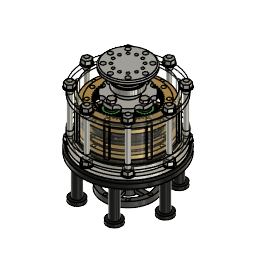
DualStagePlanetaryGearbox_2_5D_AI_Model (Autodesk Fusion 360 design; units mm, degrees)
part number: 2026-08-16-05-24-14-088
part number: 2026-08-16-14-10-31-109
part number: 2026-08-16-14-10-31-333
part number: 2026-08-16-14-11-30-504
part number: 2026-08-16-14-11-31-335
part number: 2026-08-16-14-11-32-044
part number: 2026-08-16-14-11-32-830
part number: 2026-08-16-14-11-50-183
part number: 2026-08-16-14-13-28-663
part number: 2026-08-16-14-13-28-868
part number: 2026-08-16-14-13-29-316
part number: 2026-08-16-14-13-29-716
part number: 2026-08-16-14-14-26-011
part number: 2026-08-16-14-14-26-279
part number: 2026-08-16-14-14-26-987
part number: 2026-08-16-14-14-27-816
part number: 2026-08-16-14-14-28-706
part number: 2026-08-16-14-14-29-780
part number: 2026-08-16-14-14-30-829
part number: 2026-08-16-14-16-16-341
part number: 2026-08-16-14-16-17-067
part number: 2026-08-16-14-16-17-350
part number: 2026-08-16-14-17-27-014
part number: 2026-08-16-14-17-28-983
part number: 2026-08-16-14-17-29-961
part number: 2026-08-16-14-17-30-254
part number: 2026-08-16-14-17-56-289
Autodesk Fusion 360 part; units mm, degrees
note: some values were not read from the file. Chosen so that the rebuilt part matches the saved one: which bodies a step acts on.
(part 1 of 5)
sketch "スケッチ1" plane through (0, 0, 0) normal (0, 0, 1) x (1, 0, 0) in component "Lower_Base_Plate"
  circle A0 centre (0, 0) radius 84
extrude "Base_Plate_Extrude" add sketch "スケッチ1" along normal blind 14 makes body 1 in component "Lower_Base_Plate"
sketch "スケッチ2" plane through (0, 0, 0) normal (0, 0, 1) x (1, 0, 0) in component "Lower_Base_Plate"
  circle A0 centre (0, 0) radius 32
extrude "Base_Center_Boss_Extrude" add sketch "スケッチ2" along normal blind 6 from surface at 14 bodies 1 in component "Lower_Base_Plate"
sketch "スケッチ3" plane through (0, 0, 0) normal (0, 0, 1) x (1, 0, 0) in component "Lower_Base_Plate"
  circle A0 centre (68, 0) radius 8
  circle A1 centre (34, 58.8897) radius 8
  circle A2 centre (-34, 58.8897) radius 8
  circle A3 centre (-68, 0) radius 8
  circle A4 centre (-34, -58.8897) radius 8
  circle A5 centre (34, -58.8897) radius 8
extrude "Base_Foot_Post_Extrude" add sketch "スケッチ3" along normal blind 56 from surface at -56 bodies 1 in component "Lower_Base_Plate"
sketch "スケッチ4" plane through (0, 0, 0) normal (0, 0, 1) x (1, 0, 0) in component "Lower_Base_Plate"
  circle A0 centre (68, 0) radius 13
  circle A1 centre (34, 58.8897) radius 13
  circle A2 centre (-34, 58.8897) radius 13
  circle A3 centre (-68, 0) radius 13
  circle A4 centre (-34, -58.8897) radius 13
  circle A5 centre (34, -58.8897) radius 13
extrude "Base_Foot_Pad_Extrude" add sketch "スケッチ4" along normal blind 6 from surface at -62 bodies 1 in component "Lower_Base_Plate"
sketch "スケッチ5" plane through (0, 0, 0) normal (0, 0, 1) x (1, 0, 0) in component "Lower_Base_Plate"
  circle A0 centre (0, 0) radius 13
extrude "Base_Center_Bore_Cut" cut sketch "スケッチ5" along normal blind 22 from surface at -1 bodies 1 in component "Lower_Base_Plate"
sketch "スケッチ6" plane through (0, 0, 0) normal (0, 0, 1) x (1, 0, 0) in component "Lower_Base_Plate"
  circle A0 centre (75, 0) radius 4.6
  circle A1 centre (53.033, 53.033) radius 4.6
  circle A2 centre (0, 75) radius 4.6
  circle A3 centre (-53.033, 53.033) radius 4.6
  circle A4 centre (-75, 0) radius 4.6
  circle A5 centre (-53.033, -53.033) radius 4.6
  circle A6 centre (0, -75) radius 4.6
  circle A7 centre (53.033, -53.033) radius 4.6
extrude "Base_TieRod_Hole_Cut" cut sketch "スケッチ6" along normal blind 16 from surface at -1 bodies 1 in component "Lower_Base_Plate"
sketch "スケッチ7" plane through (0, 0, 0) normal (0, 0, 1) x (1, 0, 0) in component "Lower_Base_Plate"
  circle A0 centre (48.0417, 19.8995) radius 9
  circle A1 centre (19.8995, 48.0417) radius 9
  circle A2 centre (-19.8995, 48.0417) radius 9
  circle A3 centre (-48.0417, 19.8995) radius 9
  circle A4 centre (-48.0417, -19.8995) radius 9
  circle A5 centre (-19.8995, -48.0417) radius 9
  circle A6 centre (19.8995, -48.0417) radius 9
  circle A7 centre (48.0417, -19.8995) radius 9
extrude "Base_Lightening_Hole_Cut" cut sketch "スケッチ7" along normal blind 16 from surface at -1 bodies 1 in component "Lower_Base_Plate"
sketch "スケッチ1 (2)" plane through (0, 0, 0) normal (0, 0, 1) x (1, 0, 0) in component "Lower_Housing_Ring"
  circle A0 centre (0, 0) radius 72
extrude "Housing_Ring_Extrude" add sketch "スケッチ1 (2)" along normal blind 16 from surface at 14 separate body makes body 2 in component "Lower_Housing_Ring"
sketch "スケッチ2 (2)" plane through (0, 0, 0) normal (0, 0, 1) x (1, 0, 0) in component "Lower_Housing_Ring"
  circle A0 centre (0, 0) radius 80
extrude "Housing_Ring_Flange_Extrude" add sketch "スケッチ2 (2)" along normal blind 6 from surface at 14 bodies 2 in component "Lower_Housing_Ring"
sketch "スケッチ3 (2)" plane through (0, 0, 0) normal (0, 0, 1) x (1, 0, 0) in component "Lower_Housing_Ring"
  circle A0 centre (0, 0) radius 64
extrude "Housing_Ring_Bore_Cut" cut sketch "スケッチ3 (2)" along normal blind 18 from surface at 13 bodies 2 in component "Lower_Housing_Ring"
sketch "スケッチ4 (2)" plane through (0, 0, 0) normal (0, 0, 1) x (1, 0, 0) in component "Lower_Housing_Ring"
  circle A0 centre (0, 0) radius 68
extrude "Housing_Ring_Top_Step_Cut" cut sketch "スケッチ4 (2)" along normal blind 4 from surface at 27 bodies 2 in component "Lower_Housing_Ring"
sketch "スケッチ5 (2)" plane through (0, 0, 0) normal (0, 0, 1) x (1, 0, 0) in component "Lower_Housing_Ring"
  circle A0 centre (75, 0) radius 4.6
  circle A1 centre (53.033, 53.033) radius 4.6
  circle A2 centre (0, 75) radius 4.6
  circle A3 centre (-53.033, 53.033) radius 4.6
  circle A4 centre (-75, 0) radius 4.6
  circle A5 centre (-53.033, -53.033) radius 4.6
  circle A6 centre (0, -75) radius 4.6
  circle A7 centre (53.033, -53.033) radius 4.6
extrude "Housing_Flange_Bolt_Hole_Cut" cut sketch "スケッチ5 (2)" along normal blind 8 from surface at 13 bodies 2 in component "Lower_Housing_Ring"
sketch "スケッチ1 (3)" plane through (0, 0, 0) normal (0, 0, 1) x (1, 0, 0) in component "Stage1_Sun_Gear"
  line L0 (16.0751, -1.2675) -> (16.8621, -1.3296)
  line L1 (16.8621, -1.3296) -> (17.7351, -1.2093)
  line L2 (17.7351, -1.2093) -> (18.6155, -0.9191)
  line L3 (18.6155, -0.9191) -> (19.4935, -0.5041)
  line L4 (19.4935, -0.5041) -> (19.4935, 0.5041)
  line L5 (19.4935, 0.5041) -> (18.6155, 0.9191)
  line L6 (18.6155, 0.9191) -> (17.7351, 1.2093)
  line L7 (17.7351, 1.2093) -> (16.8621, 1.3296)
  line L8 (16.8621, 1.3296) -> (16.0751, 1.2675)
  line L9 (16.0751, 1.2675) -> (15.987, 2.1047)
  line L10 (15.987, 2.1047) -> (15.8554, 2.9362)
  line L11 (15.8554, 2.9362) -> (16.6317, 3.08)
  line L12 (16.6317, 3.08) -> (17.4438, 3.422)
  line L13 (17.4438, 3.422) -> (18.2191, 3.9303)
  line L14 (18.2191, 3.9303) -> (18.9597, 4.5584)
  line L15 (18.9597, 4.5584) -> (18.6988, 5.5322)
  line L16 (18.6988, 5.5322) -> (17.7433, 5.7058)
  line L17 (17.7433, 5.7058) -> (16.8178, 5.7583)
  line L18 (16.8178, 5.7583) -> (15.9434, 5.6485)
  line L19 (15.9434, 5.6485) -> (15.1993, 5.3849)
  line L20 (15.1993, 5.3849) -> (14.8976, 6.1708)
  line L21 (14.8976, 6.1708) -> (14.5552, 6.9398)
  line L22 (14.5552, 6.9398) -> (15.2678, 7.2796)
  line L23 (15.2678, 7.2796) -> (15.9637, 7.8202)
  line L24 (15.9637, 7.8202) -> (16.581, 8.5118)
  line L25 (16.581, 8.5118) -> (17.1339, 9.3102)
  line L26 (17.1339, 9.3102) -> (16.6298, 10.1833)
  line L27 (16.6298, 10.1833) -> (15.6619, 10.1037)
  line L28 (15.6619, 10.1037) -> (14.7544, 9.9149)
  line L29 (14.7544, 9.9149) -> (13.9382, 9.5825)
  line L30 (13.9382, 9.5825) -> (13.2877, 9.1353)
  line L31 (13.2877, 9.1353) -> (12.7928, 9.8163)
  line L32 (12.7928, 9.8163) -> (12.2631, 10.4705)
  line L33 (12.2631, 10.4705) -> (12.8635, 10.9832)
  line L34 (12.8635, 10.9832) -> (13.3958, 11.6855)
  line L35 (13.3958, 11.6855) -> (13.813, 12.5132)
  line L36 (13.813, 12.5132) -> (14.1404, 13.4275)
  line L37 (14.1404, 13.4275) -> (13.4275, 14.1404)
  line L38 (13.4275, 14.1404) -> (12.5132, 13.813)
  line L39 (12.5132, 13.813) -> (11.6855, 13.3958)
  line L40 (11.6855, 13.3958) -> (10.9832, 12.8635)
  line L41 (10.9832, 12.8635) -> (10.4705, 12.2631)
  line L42 (10.4705, 12.2631) -> (9.8163, 12.7928)
  line L43 (9.8163, 12.7928) -> (9.1353, 13.2877)
  line L44 (9.1353, 13.2877) -> (9.5825, 13.9382)
  line L45 (9.5825, 13.9382) -> (9.9149, 14.7544)
  line L46 (9.9149, 14.7544) -> (10.1037, 15.6619)
  line L47 (10.1037, 15.6619) -> (10.1833, 16.6298)
  line L48 (10.1833, 16.6298) -> (9.3102, 17.1339)
  line L49 (9.3102, 17.1339) -> (8.5118, 16.581)
  line L50 (8.5118, 16.581) -> (7.8202, 15.9637)
  line L51 (7.8202, 15.9637) -> (7.2796, 15.2678)
  line L52 (7.2796, 15.2678) -> (6.9398, 14.5552)
  line L53 (6.9398, 14.5552) -> (6.1708, 14.8976)
  line L54 (6.1708, 14.8976) -> (5.3849, 15.1993)
  line L55 (5.3849, 15.1993) -> (5.6485, 15.9434)
  line L56 (5.6485, 15.9434) -> (5.7583, 16.8178)
  line L57 (5.7583, 16.8178) -> (5.7058, 17.7433)
  line L58 (5.7058, 17.7433) -> (5.5322, 18.6988)
  line L59 (5.5322, 18.6988) -> (4.5584, 18.9597)
  line L60 (4.5584, 18.9597) -> (3.9303, 18.2191)
  line L61 (3.9303, 18.2191) -> (3.422, 17.4438)
  line L62 (3.422, 17.4438) -> (3.08, 16.6317)
  line L63 (3.08, 16.6317) -> (2.9362, 15.8554)
  line L64 (2.9362, 15.8554) -> (2.1047, 15.987)
  line L65 (2.1047, 15.987) -> (1.2675, 16.0751)
  line L66 (1.2675, 16.0751) -> (1.3296, 16.8621)
  line L67 (1.3296, 16.8621) -> (1.2093, 17.7351)
  line L68 (1.2093, 17.7351) -> (0.9191, 18.6155)
  line L69 (0.9191, 18.6155) -> (0.5041, 19.4935)
  line L70 (0.5041, 19.4935) -> (-0.5041, 19.4935)
  line L71 (-0.5041, 19.4935) -> (-0.9191, 18.6155)
  line L72 (-0.9191, 18.6155) -> (-1.2093, 17.7351)
  line L73 (-1.2093, 17.7351) -> (-1.3296, 16.8621)
  line L74 (-1.3296, 16.8621) -> (-1.2675, 16.0751)
  line L75 (-1.2675, 16.0751) -> (-2.1047, 15.987)
  line L76 (-2.1047, 15.987) -> (-2.9362, 15.8554)
  line L77 (-2.9362, 15.8554) -> (-3.08, 16.6317)
  line L78 (-3.08, 16.6317) -> (-3.422, 17.4438)
  line L79 (-3.422, 17.4438) -> (-3.9303, 18.2191)
  line L80 (-3.9303, 18.2191) -> (-4.5584, 18.9597)
  line L81 (-4.5584, 18.9597) -> (-5.5322, 18.6988)
  line L82 (-5.5322, 18.6988) -> (-5.7058, 17.7433)
  line L83 (-5.7058, 17.7433) -> (-5.7583, 16.8178)
  line L84 (-5.7583, 16.8178) -> (-5.6485, 15.9434)
  line L85 (-5.6485, 15.9434) -> (-5.3849, 15.1993)
  line L86 (-5.3849, 15.1993) -> (-6.1708, 14.8976)
  line L87 (-6.1708, 14.8976) -> (-6.9398, 14.5552)
  line L88 (-6.9398, 14.5552) -> (-7.2796, 15.2678)
  line L89 (-7.2796, 15.2678) -> (-7.8202, 15.9637)
  line L90 (-7.8202, 15.9637) -> (-8.5118, 16.581)
  line L91 (-8.5118, 16.581) -> (-9.3102, 17.1339)
  line L92 (-9.3102, 17.1339) -> (-10.1833, 16.6298)
  line L93 (-10.1833, 16.6298) -> (-10.1037, 15.6619)
  line L94 (-10.1037, 15.6619) -> (-9.9149, 14.7544)
  line L95 (-9.9149, 14.7544) -> (-9.5825, 13.9382)
  line L96 (-9.5825, 13.9382) -> (-9.1353, 13.2877)
  line L97 (-9.1353, 13.2877) -> (-9.8163, 12.7928)
  line L98 (-9.8163, 12.7928) -> (-10.4705, 12.2631)
  line L99 (-10.4705, 12.2631) -> (-10.9832, 12.8635)
  line L100 (-10.9832, 12.8635) -> (-11.6855, 13.3958)
  line L101 (-11.6855, 13.3958) -> (-12.5132, 13.813)
  line L102 (-12.5132, 13.813) -> (-13.4275, 14.1404)
  line L103 (-13.4275, 14.1404) -> (-14.1404, 13.4275)
  line L104 (-14.1404, 13.4275) -> (-13.813, 12.5132)
  line L105 (-13.813, 12.5132) -> (-13.3958, 11.6855)
  line L106 (-13.3958, 11.6855) -> (-12.8635, 10.9832)
  line L107 (-12.8635, 10.9832) -> (-12.2631, 10.4705)
  line L108 (-12.2631, 10.4705) -> (-12.7928, 9.8163)
  line L109 (-12.7928, 9.8163) -> (-13.2877, 9.1353)
  line L110 (-13.2877, 9.1353) -> (-13.9382, 9.5825)
  line L111 (-13.9382, 9.5825) -> (-14.7544, 9.9149)
  line L112 (-14.7544, 9.9149) -> (-15.6619, 10.1037)
  line L113 (-15.6619, 10.1037) -> (-16.6298, 10.1833)
  line L114 (-16.6298, 10.1833) -> (-17.1339, 9.3102)
  line L115 (-17.1339, 9.3102) -> (-16.581, 8.5118)
  line L116 (-16.581, 8.5118) -> (-15.9637, 7.8202)
  line L117 (-15.9637, 7.8202) -> (-15.2678, 7.2796)
  line L118 (-15.2678, 7.2796) -> (-14.5552, 6.9398)
  line L119 (-14.5552, 6.9398) -> (-14.8976, 6.1708)
  line L120 (-14.8976, 6.1708) -> (-15.1993, 5.3849)
  line L121 (-15.1993, 5.3849) -> (-15.9434, 5.6485)
  line L122 (-15.9434, 5.6485) -> (-16.8178, 5.7583)
  line L123 (-16.8178, 5.7583) -> (-17.7433, 5.7058)
  line L124 (-17.7433, 5.7058) -> (-18.6988, 5.5322)
  line L125 (-18.6988, 5.5322) -> (-18.9597, 4.5584)
  line L126 (-18.9597, 4.5584) -> (-18.2191, 3.9303)
  line L127 (-18.2191, 3.9303) -> (-17.4438, 3.422)
  line L128 (-17.4438, 3.422) -> (-16.6317, 3.08)
  line L129 (-16.6317, 3.08) -> (-15.8554, 2.9362)
  line L130 (-15.8554, 2.9362) -> (-15.987, 2.1047)
  line L131 (-15.987, 2.1047) -> (-16.0751, 1.2675)
  line L132 (-16.0751, 1.2675) -> (-16.8621, 1.3296)
  line L133 (-16.8621, 1.3296) -> (-17.7351, 1.2093)
  line L134 (-17.7351, 1.2093) -> (-18.6155, 0.9191)
  line L135 (-18.6155, 0.9191) -> (-19.4935, 0.5041)
  line L136 (-19.4935, 0.5041) -> (-19.4935, -0.5041)
  line L137 (-19.4935, -0.5041) -> (-18.6155, -0.9191)
  line L138 (-18.6155, -0.9191) -> (-17.7351, -1.2093)
  line L139 (-17.7351, -1.2093) -> (-16.8621, -1.3296)
  line L140 (-16.8621, -1.3296) -> (-16.0751, -1.2675)
  line L141 (-16.0751, -1.2675) -> (-15.987, -2.1047)
  line L142 (-15.987, -2.1047) -> (-15.8554, -2.9362)
  line L143 (-15.8554, -2.9362) -> (-16.6317, -3.08)
  line L144 (-16.6317, -3.08) -> (-17.4438, -3.422)
  line L145 (-17.4438, -3.422) -> (-18.2191, -3.9303)
  line L146 (-18.2191, -3.9303) -> (-18.9597, -4.5584)
  line L147 (-18.9597, -4.5584) -> (-18.6988, -5.5322)
  line L148 (-18.6988, -5.5322) -> (-17.7433, -5.7058)
  line L149 (-17.7433, -5.7058) -> (-16.8178, -5.7583)
  line L150 (-16.8178, -5.7583) -> (-15.9434, -5.6485)
  line L151 (-15.9434, -5.6485) -> (-15.1993, -5.3849)
  line L152 (-15.1993, -5.3849) -> (-14.8976, -6.1708)
  line L153 (-14.8976, -6.1708) -> (-14.5552, -6.9398)
  line L154 (-14.5552, -6.9398) -> (-15.2678, -7.2796)
  line L155 (-15.2678, -7.2796) -> (-15.9637, -7.8202)
  line L156 (-15.9637, -7.8202) -> (-16.581, -8.5118)
  line L157 (-16.581, -8.5118) -> (-17.1339, -9.3102)
  line L158 (-17.1339, -9.3102) -> (-16.6298, -10.1833)
  line L159 (-16.6298, -10.1833) -> (-15.6619, -10.1037)
  line L160 (-15.6619, -10.1037) -> (-14.7544, -9.9149)
  line L161 (-14.7544, -9.9149) -> (-13.9382, -9.5825)
  line L162 (-13.9382, -9.5825) -> (-13.2877, -9.1353)
  line L163 (-13.2877, -9.1353) -> (-12.7928, -9.8163)
  line L164 (-12.7928, -9.8163) -> (-12.2631, -10.4705)
  line L165 (-12.2631, -10.4705) -> (-12.8635, -10.9832)
  line L166 (-12.8635, -10.9832) -> (-13.3958, -11.6855)
  line L167 (-13.3958, -11.6855) -> (-13.813, -12.5132)
  line L168 (-13.813, -12.5132) -> (-14.1404, -13.4275)
  line L169 (-14.1404, -13.4275) -> (-13.4275, -14.1404)
  line L170 (-13.4275, -14.1404) -> (-12.5132, -13.813)
  line L171 (-12.5132, -13.813) -> (-11.6855, -13.3958)
  line L172 (-11.6855, -13.3958) -> (-10.9832, -12.8635)
  line L173 (-10.9832, -12.8635) -> (-10.4705, -12.2631)
  line L174 (-10.4705, -12.2631) -> (-9.8163, -12.7928)
  line L175 (-9.8163, -12.7928) -> (-9.1353, -13.2877)
  line L176 (-9.1353, -13.2877) -> (-9.5825, -13.9382)
  line L177 (-9.5825, -13.9382) -> (-9.9149, -14.7544)
  line L178 (-9.9149, -14.7544) -> (-10.1037, -15.6619)
  line L179 (-10.1037, -15.6619) -> (-10.1833, -16.6298)
  line L180 (-10.1833, -16.6298) -> (-9.3102, -17.1339)
  line L181 (-9.3102, -17.1339) -> (-8.5118, -16.581)
  line L182 (-8.5118, -16.581) -> (-7.8202, -15.9637)
  line L183 (-7.8202, -15.9637) -> (-7.2796, -15.2678)
  line L184 (-7.2796, -15.2678) -> (-6.9398, -14.5552)
  line L185 (-6.9398, -14.5552) -> (-6.1708, -14.8976)
  line L186 (-6.1708, -14.8976) -> (-5.3849, -15.1993)
  line L187 (-5.3849, -15.1993) -> (-5.6485, -15.9434)
  line L188 (-5.6485, -15.9434) -> (-5.7583, -16.8178)
  line L189 (-5.7583, -16.8178) -> (-5.7058, -17.7433)
  line L190 (-5.7058, -17.7433) -> (-5.5322, -18.6988)
  line L191 (-5.5322, -18.6988) -> (-4.5584, -18.9597)
  line L192 (-4.5584, -18.9597) -> (-3.9303, -18.2191)
  line L193 (-3.9303, -18.2191) -> (-3.422, -17.4438)
  line L194 (-3.422, -17.4438) -> (-3.08, -16.6317)
  line L195 (-3.08, -16.6317) -> (-2.9362, -15.8554)
  line L196 (-2.9362, -15.8554) -> (-2.1047, -15.987)
  line L197 (-2.1047, -15.987) -> (-1.2675, -16.0751)
  line L198 (-1.2675, -16.0751) -> (-1.3296, -16.8621)
  line L199 (-1.3296, -16.8621) -> (-1.2093, -17.7351)
  line L200 (-1.2093, -17.7351) -> (-0.9191, -18.6155)
  line L201 (-0.9191, -18.6155) -> (-0.5041, -19.4935)
  line L202 (-0.5041, -19.4935) -> (0.5041, -19.4935)
  line L203 (0.5041, -19.4935) -> (0.9191, -18.6155)
  line L204 (0.9191, -18.6155) -> (1.2093, -17.7351)
  line L205 (1.2093, -17.7351) -> (1.3296, -16.8621)
  line L206 (1.3296, -16.8621) -> (1.2675, -16.0751)
  line L207 (1.2675, -16.0751) -> (2.1047, -15.987)
  line L208 (2.1047, -15.987) -> (2.9362, -15.8554)
  line L209 (2.9362, -15.8554) -> (3.08, -16.6317)
  line L210 (3.08, -16.6317) -> (3.422, -17.4438)
  line L211 (3.422, -17.4438) -> (3.9303, -18.2191)
  line L212 (3.9303, -18.2191) -> (4.5584, -18.9597)
  line L213 (4.5584, -18.9597) -> (5.5322, -18.6988)
  line L214 (5.5322, -18.6988) -> (5.7058, -17.7433)
  line L215 (5.7058, -17.7433) -> (5.7583, -16.8178)
  line L216 (5.7583, -16.8178) -> (5.6485, -15.9434)
  line L217 (5.6485, -15.9434) -> (5.3849, -15.1993)
  line L218 (5.3849, -15.1993) -> (6.1708, -14.8976)
  line L219 (6.1708, -14.8976) -> (6.9398, -14.5552)
  line L220 (6.9398, -14.5552) -> (7.2796, -15.2678)
  line L221 (7.2796, -15.2678) -> (7.8202, -15.9637)
  line L222 (7.8202, -15.9637) -> (8.5118, -16.581)
  line L223 (8.5118, -16.581) -> (9.3102, -17.1339)
  line L224 (9.3102, -17.1339) -> (10.1833, -16.6298)
  line L225 (10.1833, -16.6298) -> (10.1037, -15.6619)
  line L226 (10.1037, -15.6619) -> (9.9149, -14.7544)
  line L227 (9.9149, -14.7544) -> (9.5825, -13.9382)
  line L228 (9.5825, -13.9382) -> (9.1353, -13.2877)
  line L229 (9.1353, -13.2877) -> (9.8163, -12.7928)
  line L230 (9.8163, -12.7928) -> (10.4705, -12.2631)
  line L231 (10.4705, -12.2631) -> (10.9832, -12.8635)
  line L232 (10.9832, -12.8635) -> (11.6855, -13.3958)
  line L233 (11.6855, -13.3958) -> (12.5132, -13.813)
  line L234 (12.5132, -13.813) -> (13.4275, -14.1404)
  line L235 (13.4275, -14.1404) -> (14.1404, -13.4275)
  line L236 (14.1404, -13.4275) -> (13.813, -12.5132)
  line L237 (13.813, -12.5132) -> (13.3958, -11.6855)
  line L238 (13.3958, -11.6855) -> (12.8635, -10.9832)
  line L239 (12.8635, -10.9832) -> (12.2631, -10.4705)
  line L240 (12.2631, -10.4705) -> (12.7928, -9.8163)
  line L241 (12.7928, -9.8163) -> (13.2877, -9.1353)
  line L242 (13.2877, -9.1353) -> (13.9382, -9.5825)
  line L243 (13.9382, -9.5825) -> (14.7544, -9.9149)
  line L244 (14.7544, -9.9149) -> (15.6619, -10.1037)
  line L245 (15.6619, -10.1037) -> (16.6298, -10.1833)
  line L246 (16.6298, -10.1833) -> (17.1339, -9.3102)
  line L247 (17.1339, -9.3102) -> (16.581, -8.5118)
  line L248 (16.581, -8.5118) -> (15.9637, -7.8202)
  line L249 (15.9637, -7.8202) -> (15.2678, -7.2796)
  line L250 (15.2678, -7.2796) -> (14.5552, -6.9398)
  line L251 (14.5552, -6.9398) -> (14.8976, -6.1708)
  line L252 (14.8976, -6.1708) -> (15.1993, -5.3849)
  line L253 (15.1993, -5.3849) -> (15.9434, -5.6485)
  line L254 (15.9434, -5.6485) -> (16.8178, -5.7583)
  line L255 (16.8178, -5.7583) -> (17.7433, -5.7058)
  line L256 (17.7433, -5.7058) -> (18.6988, -5.5322)
  line L257 (18.6988, -5.5322) -> (18.9597, -4.5584)
  line L258 (18.9597, -4.5584) -> (18.2191, -3.9303)
  line L259 (18.2191, -3.9303) -> (17.4438, -3.422)
  line L260 (17.4438, -3.422) -> (16.6317, -3.08)
  line L261 (16.6317, -3.08) -> (15.8554, -2.9362)
  line L262 (15.8554, -2.9362) -> (15.987, -2.1047)
  line L263 (15.987, -2.1047) -> (16.0751, -1.2675)
extrude "Stage1_Sun_Extrude" add sketch "スケッチ1 (3)" along normal blind 12 from surface at 34 separate body makes body 3 in component "Stage1_Sun_Gear"
sketch "スケッチ2 (3)" plane through (0, 0, 0) normal (0, 0, 1) x (1, 0, 0) in component "Stage1_Sun_Gear"
  circle A0 centre (0, 0) radius 15
extrude "Stage1_Sun_Hub_Lower_Extrude" add sketch "スケッチ2 (3)" along normal blind 3.5 from surface at 30.5 bodies 3 in component "Stage1_Sun_Gear"
sketch "スケッチ3 (3)" plane through (0, 0, 0) normal (0, 0, 1) x (1, 0, 0) in component "Stage1_Sun_Gear"
  circle A0 centre (0, 0) radius 11
extrude "Stage1_Sun_Hub_Upper_Extrude" add sketch "スケッチ3 (3)" along normal blind 3.5 from surface at 46 bodies 3 in component "Stage1_Sun_Gear"
sketch "スケッチ4 (3)" plane through (0, 0, 0) normal (0, 0, 1) x (1, 0, 0) in component "Stage1_Sun_Gear"
  circle A0 centre (0, 0) radius 10
extrude "Stage1_Sun_Bore_Cut" cut sketch "スケッチ4 (3)" along normal blind 22 from surface at 29 bodies 3 in component "Stage1_Sun_Gear"
sketch "スケッチ5 (3)" plane through (0, 0, 0) normal (0, 0, 1) x (1, 0, 0) in component "Stage1_Sun_Gear"
  line L0 (-3, 9) -> (3, 9)
  line L1 (3, 9) -> (3, 12.5)
  line L2 (3, 12.5) -> (-3, 12.5)
  line L3 (-3, 12.5) -> (-3, 9)
extrude "Stage1_Sun_Keyway_Cut" cut sketch "スケッチ5 (3)" along normal blind 22 from surface at 29 bodies 3 in component "Stage1_Sun_Gear"
sketch "スケッチ1 (4)" plane through (0, 0, 0) normal (0, 0, 1) x (1, 0, 0) in component "Stage1_Planet_Gear_A"
  line L0 (20.3102, 3.1509) -> (19.289, 3.4385)
  line L1 (19.289, 3.4385) -> (18.4975, 3.4689)
  line L2 (18.4975, 3.4689) -> (17.6675, 3.334)
  line L3 (17.6675, 3.334) -> (16.8184, 3.074)
  line L4 (16.8184, 3.074) -> (16.6524, 2.1328)
  line L5 (16.6524, 2.1328) -> (17.3614, 1.598)
  line L6 (17.3614, 1.598) -> (18.0953, 1.1874)
  line L7 (18.0953, 1.1874) -> (18.8494, 0.9453)
  line L8 (18.8494, 0.9453) -> (19.9073, 0.8662)
  line L9 (19.9073, 0.8662) -> (19.875, 0)
  line L10 (19.875, 0) -> (19.9073, -0.8662)
  line L11 (19.9073, -0.8662) -> (18.8494, -0.9453)
  line L12 (18.8494, -0.9453) -> (18.0953, -1.1874)
  line L13 (18.0953, -1.1874) -> (17.3614, -1.598)
  line L14 (17.3614, -1.598) -> (16.6524, -2.1328)
  line L15 (16.6524, -2.1328) -> (16.8184, -3.074)
  line L16 (16.8184, -3.074) -> (17.6675, -3.334)
  line L17 (17.6675, -3.334) -> (18.4975, -3.4689)
  line L18 (18.4975, -3.4689) -> (19.289, -3.4385)
  line L19 (19.289, -3.4385) -> (20.3102, -3.1509)
  line L20 (20.3102, -3.1509) -> (20.5761, -3.976)
  line L21 (20.5761, -3.976) -> (20.9027, -4.7789)
  line L22 (20.9027, -4.7789) -> (19.9356, -5.215)
  line L23 (19.9356, -5.215) -> (19.3098, -5.7005)
  line L24 (19.3098, -5.7005) -> (18.7606, -6.3373)
  line L25 (18.7606, -6.3373) -> (18.2773, -7.0824)
  line L26 (18.2773, -7.0824) -> (18.7551, -7.91)
  line L27 (18.7551, -7.91) -> (19.642, -7.864)
  line L28 (19.642, -7.864) -> (20.4681, -7.7068)
  line L29 (20.4681, -7.7068) -> (21.2015, -7.4075)
  line L30 (21.2015, -7.4075) -> (22.0627, -6.7881)
  line L31 (22.0627, -6.7881) -> (22.5947, -7.4724)
  line L32 (22.5947, -7.4724) -> (23.1763, -8.1152)
  line L33 (23.1763, -8.1152) -> (22.4167, -8.8558)
  line L34 (22.4167, -8.8558) -> (21.9946, -9.526)
  line L35 (21.9946, -9.526) -> (21.6964, -10.3123)
  line L36 (21.6964, -10.3123) -> (21.497, -11.1777)
  line L37 (21.497, -11.1777) -> (22.2291, -11.792)
  line L38 (22.2291, -11.792) -> (23.0468, -11.4454)
  line L39 (23.0468, -11.4454) -> (23.7693, -11.0152)
  line L40 (23.7693, -11.0152) -> (24.3561, -10.4831)
  line L41 (24.3561, -10.4831) -> (24.9535, -9.6064)
  line L42 (24.9535, -9.6064) -> (25.6875, -10.0675)
  line L43 (25.6875, -10.0675) -> (26.4538, -10.4727)
  line L44 (26.4538, -10.4727) -> (25.9934, -11.4284)
  line L45 (25.9934, -11.4284) -> (25.8259, -12.2025)
  line L46 (25.8259, -12.2025) -> (25.8146, -13.0434)
  line L47 (25.8146, -13.0434) -> (25.9233, -13.9248)
  line L48 (25.9233, -13.9248) -> (26.8213, -14.2517)
  line L49 (26.8213, -14.2517) -> (27.4711, -13.6463)
  line L50 (27.4711, -13.6463) -> (28.0029, -12.9949)
  line L51 (28.0029, -12.9949) -> (28.3723, -12.2942)
  line L52 (28.3723, -12.2942) -> (28.6339, -11.2661)
  line L53 (28.6339, -11.2661) -> (29.4813, -11.4484)
  line L54 (29.4813, -11.4484) -> (30.34, -11.567)
  line L55 (30.34, -11.567) -> (30.2342, -12.6225)
  line L56 (30.2342, -12.6225) -> (30.3416, -13.4073)
  line L57 (30.3416, -13.4073) -> (30.6186, -14.2013)
  line L58 (30.6186, -14.2013) -> (31.0222, -14.9924)
  line L59 (31.0222, -14.9924) -> (31.9778, -14.9924)
  line L60 (31.9778, -14.9924) -> (32.3814, -14.2013)
  line L61 (32.3814, -14.2013) -> (32.6584, -13.4073)
  line L62 (32.6584, -13.4073) -> (32.7658, -12.6225)
  line L63 (32.7658, -12.6225) -> (32.66, -11.567)
  line L64 (32.66, -11.567) -> (33.5187, -11.4484)
  line L65 (33.5187, -11.4484) -> (34.3661, -11.2661)
  line L66 (34.3661, -11.2661) -> (34.6277, -12.2942)
  line L67 (34.6277, -12.2942) -> (34.9971, -12.9949)
  line L68 (34.9971, -12.9949) -> (35.5289, -13.6463)
  line L69 (35.5289, -13.6463) -> (36.1787, -14.2517)
  line L70 (36.1787, -14.2517) -> (37.0767, -13.9248)
  line L71 (37.0767, -13.9248) -> (37.1854, -13.0434)
  line L72 (37.1854, -13.0434) -> (37.1741, -12.2025)
  line L73 (37.1741, -12.2025) -> (37.0066, -11.4284)
  line L74 (37.0066, -11.4284) -> (36.5462, -10.4727)
  line L75 (36.5462, -10.4727) -> (37.3125, -10.0675)
  line L76 (37.3125, -10.0675) -> (38.0465, -9.6064)
  line L77 (38.0465, -9.6064) -> (38.6439, -10.4831)
  line L78 (38.6439, -10.4831) -> (39.2307, -11.0152)
  line L79 (39.2307, -11.0152) -> (39.9532, -11.4454)
  line L80 (39.9532, -11.4454) -> (40.7709, -11.792)
  line L81 (40.7709, -11.792) -> (41.503, -11.1777)
  line L82 (41.503, -11.1777) -> (41.3036, -10.3123)
  line L83 (41.3036, -10.3123) -> (41.0054, -9.526)
  line L84 (41.0054, -9.526) -> (40.5833, -8.8558)
  line L85 (40.5833, -8.8558) -> (39.8237, -8.1152)
  line L86 (39.8237, -8.1152) -> (40.4053, -7.4724)
  line L87 (40.4053, -7.4724) -> (40.9373, -6.7881)
  line L88 (40.9373, -6.7881) -> (41.7985, -7.4075)
  line L89 (41.7985, -7.4075) -> (42.5319, -7.7068)
  line L90 (42.5319, -7.7068) -> (43.358, -7.864)
  line L91 (43.358, -7.864) -> (44.2449, -7.91)
  line L92 (44.2449, -7.91) -> (44.7227, -7.0824)
  line L93 (44.7227, -7.0824) -> (44.2394, -6.3373)
  line L94 (44.2394, -6.3373) -> (43.6902, -5.7005)
  line L95 (43.6902, -5.7005) -> (43.0644, -5.215)
  line L96 (43.0644, -5.215) -> (42.0973, -4.7789)
  line L97 (42.0973, -4.7789) -> (42.4239, -3.976)
  line L98 (42.4239, -3.976) -> (42.6898, -3.1509)
  line L99 (42.6898, -3.1509) -> (43.711, -3.4385)
  line L100 (43.711, -3.4385) -> (44.5025, -3.4689)
  line L101 (44.5025, -3.4689) -> (45.3325, -3.334)
  line L102 (45.3325, -3.334) -> (46.1816, -3.074)
  line L103 (46.1816, -3.074) -> (46.3476, -2.1328)
  line L104 (46.3476, -2.1328) -> (45.6386, -1.598)
  line L105 (45.6386, -1.598) -> (44.9047, -1.1874)
  line L106 (44.9047, -1.1874) -> (44.1506, -0.9453)
  line L107 (44.1506, -0.9453) -> (43.0927, -0.8662)
  line L108 (43.0927, -0.8662) -> (43.125, 0)
  line L109 (43.125, 0) -> (43.0927, 0.8662)
  line L110 (43.0927, 0.8662) -> (44.1506, 0.9453)
  line L111 (44.1506, 0.9453) -> (44.9047, 1.1874)
  line L112 (44.9047, 1.1874) -> (45.6386, 1.598)
  line L113 (45.6386, 1.598) -> (46.3476, 2.1328)
  line L114 (46.3476, 2.1328) -> (46.1816, 3.074)
  line L115 (46.1816, 3.074) -> (45.3325, 3.334)
  line L116 (45.3325, 3.334) -> (44.5025, 3.4689)
  line L117 (44.5025, 3.4689) -> (43.711, 3.4385)
  line L118 (43.711, 3.4385) -> (42.6898, 3.1509)
  line L119 (42.6898, 3.1509) -> (42.4239, 3.976)
  line L120 (42.4239, 3.976) -> (42.0973, 4.7789)
  line L121 (42.0973, 4.7789) -> (43.0644, 5.215)
  line L122 (43.0644, 5.215) -> (43.6902, 5.7005)
  line L123 (43.6902, 5.7005) -> (44.2394, 6.3373)
  line L124 (44.2394, 6.3373) -> (44.7227, 7.0824)
  line L125 (44.7227, 7.0824) -> (44.2449, 7.91)
  line L126 (44.2449, 7.91) -> (43.358, 7.864)
  line L127 (43.358, 7.864) -> (42.5319, 7.7068)
  line L128 (42.5319, 7.7068) -> (41.7985, 7.4075)
  line L129 (41.7985, 7.4075) -> (40.9373, 6.7881)
  line L130 (40.9373, 6.7881) -> (40.4053, 7.4724)
  line L131 (40.4053, 7.4724) -> (39.8237, 8.1152)
  line L132 (39.8237, 8.1152) -> (40.5833, 8.8558)
  line L133 (40.5833, 8.8558) -> (41.0054, 9.526)
  line L134 (41.0054, 9.526) -> (41.3036, 10.3123)
  line L135 (41.3036, 10.3123) -> (41.503, 11.1777)
  line L136 (41.503, 11.1777) -> (40.7709, 11.792)
  line L137 (40.7709, 11.792) -> (39.9532, 11.4454)
  line L138 (39.9532, 11.4454) -> (39.2307, 11.0152)
  line L139 (39.2307, 11.0152) -> (38.6439, 10.4831)
  line L140 (38.6439, 10.4831) -> (38.0465, 9.6064)
  line L141 (38.0465, 9.6064) -> (37.3125, 10.0675)
  line L142 (37.3125, 10.0675) -> (36.5462, 10.4727)
  line L143 (36.5462, 10.4727) -> (37.0066, 11.4284)
  line L144 (37.0066, 11.4284) -> (37.1741, 12.2025)
  line L145 (37.1741, 12.2025) -> (37.1854, 13.0434)
  line L146 (37.1854, 13.0434) -> (37.0767, 13.9248)
  line L147 (37.0767, 13.9248) -> (36.1787, 14.2517)
  line L148 (36.1787, 14.2517) -> (35.5289, 13.6463)
  line L149 (35.5289, 13.6463) -> (34.9971, 12.9949)
  line L150 (34.9971, 12.9949) -> (34.6277, 12.2942)
  line L151 (34.6277, 12.2942) -> (34.3661, 11.2661)
  line L152 (34.3661, 11.2661) -> (33.5187, 11.4484)
  line L153 (33.5187, 11.4484) -> (32.66, 11.567)
  line L154 (32.66, 11.567) -> (32.7658, 12.6225)
  line L155 (32.7658, 12.6225) -> (32.6584, 13.4073)
  line L156 (32.6584, 13.4073) -> (32.3814, 14.2013)
  line L157 (32.3814, 14.2013) -> (31.9778, 14.9924)
  line L158 (31.9778, 14.9924) -> (31.0222, 14.9924)
  line L159 (31.0222, 14.9924) -> (30.6186, 14.2013)
  line L160 (30.6186, 14.2013) -> (30.3416, 13.4073)
  line L161 (30.3416, 13.4073) -> (30.2342, 12.6225)
  line L162 (30.2342, 12.6225) -> (30.34, 11.567)
  line L163 (30.34, 11.567) -> (29.4813, 11.4484)
  line L164 (29.4813, 11.4484) -> (28.6339, 11.2661)
  line L165 (28.6339, 11.2661) -> (28.3723, 12.2942)
  line L166 (28.3723, 12.2942) -> (28.0029, 12.9949)
  line L167 (28.0029, 12.9949) -> (27.4711, 13.6463)
  line L168 (27.4711, 13.6463) -> (26.8213, 14.2517)
  line L169 (26.8213, 14.2517) -> (25.9233, 13.9248)
  line L170 (25.9233, 13.9248) -> (25.8146, 13.0434)
  line L171 (25.8146, 13.0434) -> (25.8259, 12.2025)
  line L172 (25.8259, 12.2025) -> (25.9934, 11.4284)
  line L173 (25.9934, 11.4284) -> (26.4538, 10.4727)
  line L174 (26.4538, 10.4727) -> (25.6875, 10.0675)
  line L175 (25.6875, 10.0675) -> (24.9535, 9.6064)
  line L176 (24.9535, 9.6064) -> (24.3561, 10.4831)
  line L177 (24.3561, 10.4831) -> (23.7693, 11.0152)
  line L178 (23.7693, 11.0152) -> (23.0468, 11.4454)
  line L179 (23.0468, 11.4454) -> (22.2291, 11.792)
  line L180 (22.2291, 11.792) -> (21.497, 11.1777)
  line L181 (21.497, 11.1777) -> (21.6964, 10.3123)
  line L182 (21.6964, 10.3123) -> (21.9946, 9.526)
  line L183 (21.9946, 9.526) -> (22.4167, 8.8558)
  line L184 (22.4167, 8.8558) -> (23.1763, 8.1152)
  line L185 (23.1763, 8.1152) -> (22.5947, 7.4724)
  line L186 (22.5947, 7.4724) -> (22.0627, 6.7881)
  line L187 (22.0627, 6.7881) -> (21.2015, 7.4075)
  line L188 (21.2015, 7.4075) -> (20.4681, 7.7068)
  line L189 (20.4681, 7.7068) -> (19.642, 7.864)
  line L190 (19.642, 7.864) -> (18.7551, 7.91)
  line L191 (18.7551, 7.91) -> (18.2773, 7.0824)
  line L192 (18.2773, 7.0824) -> (18.7606, 6.3373)
  line L193 (18.7606, 6.3373) -> (19.3098, 5.7005)
  line L194 (19.3098, 5.7005) -> (19.9356, 5.215)
  line L195 (19.9356, 5.215) -> (20.9027, 4.7789)
  line L196 (20.9027, 4.7789) -> (20.5761, 3.976)
  line L197 (20.5761, 3.976) -> (20.3102, 3.1509)
extrude "Stage1_Planet_A_Extrude" add sketch "スケッチ1 (4)" along normal blind 12 from surface at 34 separate body makes body 4 in component "Stage1_Planet_Gear_A"
sketch "スケッチ2 (4)" plane through (0, 0, 0) normal (0, 0, 1) x (1, 0, 0) in component "Stage1_Planet_Gear_A"
  circle A0 centre (31.5, 0) radius 8
extrude "Stage1_Planet_A_Hub_Lower_Extrude" add sketch "スケッチ2 (4)" along normal blind 3.5 from surface at 30.5 bodies 4 in component "Stage1_Planet_Gear_A"
sketch "スケッチ3 (4)" plane through (0, 0, 0) normal (0, 0, 1) x (1, 0, 0) in component "Stage1_Planet_Gear_A"
  circle A0 centre (31.5, 0) radius 8
extrude "Stage1_Planet_A_Hub_Upper_Extrude" add sketch "スケッチ3 (4)" along normal blind 3.5 from surface at 46 bodies 4 in component "Stage1_Planet_Gear_A"
sketch "スケッチ4 (4)" plane through (0, 0, 0) normal (0, 0, 1) x (1, 0, 0) in component "Stage1_Planet_Gear_A"
  circle A0 centre (31.5, 0) radius 4.3
extrude "Stage1_Planet_A_Bore_Cut" cut sketch "スケッチ4 (4)" along normal blind 22 from surface at 29 bodies 4 in component "Stage1_Planet_Gear_A"
sketch "スケッチ1 (5)" plane through (0, 0, 0) normal (0, 0, 1) x (1, 0, 0) in component "Stage1_Planet_Gear_B"
  line L0 (-22.2965, 36.8862) -> (-22.8939, 37.7629)
  line L1 (-22.8939, 37.7629) -> (-23.4807, 38.295)
  line L2 (-23.4807, 38.295) -> (-24.2032, 38.7252)
  line L3 (-24.2032, 38.7252) -> (-25.0209, 39.0718)
  line L4 (-25.0209, 39.0718) -> (-25.753, 38.4575)
  line L5 (-25.753, 38.4575) -> (-25.5536, 37.5921)
  line L6 (-25.5536, 37.5921) -> (-25.2554, 36.8058)
  line L7 (-25.2554, 36.8058) -> (-24.8333, 36.1356)
  line L8 (-24.8333, 36.1356) -> (-24.0737, 35.395)
  line L9 (-24.0737, 35.395) -> (-24.6553, 34.7522)
  line L10 (-24.6553, 34.7522) -> (-25.1873, 34.0679)
  line L11 (-25.1873, 34.0679) -> (-26.0485, 34.6873)
  line L12 (-26.0485, 34.6873) -> (-26.7819, 34.9866)
  line L13 (-26.7819, 34.9866) -> (-27.608, 35.1438)
  line L14 (-27.608, 35.1438) -> (-28.4949, 35.1898)
  line L15 (-28.4949, 35.1898) -> (-28.9727, 34.3622)
  line L16 (-28.9727, 34.3622) -> (-28.4894, 33.6171)
  line L17 (-28.4894, 33.6171) -> (-27.9402, 32.9803)
  line L18 (-27.9402, 32.9803) -> (-27.3144, 32.4948)
  line L19 (-27.3144, 32.4948) -> (-26.3473, 32.0587)
  line L20 (-26.3473, 32.0587) -> (-26.6739, 31.2558)
  line L21 (-26.6739, 31.2558) -> (-26.9398, 30.4307)
  line L22 (-26.9398, 30.4307) -> (-27.961, 30.7183)
  line L23 (-27.961, 30.7183) -> (-28.7525, 30.7487)
  line L24 (-28.7525, 30.7487) -> (-29.5825, 30.6138)
  line L25 (-29.5825, 30.6138) -> (-30.4316, 30.3538)
  line L26 (-30.4316, 30.3538) -> (-30.5976, 29.4126)
  line L27 (-30.5976, 29.4126) -> (-29.8886, 28.8778)
  line L28 (-29.8886, 28.8778) -> (-29.1547, 28.4672)
  line L29 (-29.1547, 28.4672) -> (-28.4006, 28.2251)
  line L30 (-28.4006, 28.2251) -> (-27.3427, 28.146)
  line L31 (-27.3427, 28.146) -> (-27.375, 27.2798)
  line L32 (-27.375, 27.2798) -> (-27.3427, 26.4136)
  line L33 (-27.3427, 26.4136) -> (-28.4006, 26.3345)
  line L34 (-28.4006, 26.3345) -> (-29.1547, 26.0924)
  line L35 (-29.1547, 26.0924) -> (-29.8886, 25.6818)
  line L36 (-29.8886, 25.6818) -> (-30.5976, 25.147)
  line L37 (-30.5976, 25.147) -> (-30.4316, 24.2058)
  line L38 (-30.4316, 24.2058) -> (-29.5825, 23.9458)
  line L39 (-29.5825, 23.9458) -> (-28.7525, 23.8109)
  line L40 (-28.7525, 23.8109) -> (-27.961, 23.8413)
  line L41 (-27.961, 23.8413) -> (-26.9398, 24.1289)
  line L42 (-26.9398, 24.1289) -> (-26.6739, 23.3038)
  line L43 (-26.6739, 23.3038) -> (-26.3473, 22.5009)
  line L44 (-26.3473, 22.5009) -> (-27.3144, 22.0648)
  line L45 (-27.3144, 22.0648) -> (-27.9402, 21.5793)
  line L46 (-27.9402, 21.5793) -> (-28.4894, 20.9425)
  line L47 (-28.4894, 20.9425) -> (-28.9727, 20.1974)
  line L48 (-28.9727, 20.1974) -> (-28.4949, 19.3698)
  line L49 (-28.4949, 19.3698) -> (-27.608, 19.4158)
  line L50 (-27.608, 19.4158) -> (-26.7819, 19.573)
  line L51 (-26.7819, 19.573) -> (-26.0485, 19.8723)
  line L52 (-26.0485, 19.8723) -> (-25.1873, 20.4917)
  line L53 (-25.1873, 20.4917) -> (-24.6553, 19.8074)
  line L54 (-24.6553, 19.8074) -> (-24.0737, 19.1646)
  line L55 (-24.0737, 19.1646) -> (-24.8333, 18.424)
  line L56 (-24.8333, 18.424) -> (-25.2554, 17.7538)
  line L57 (-25.2554, 17.7538) -> (-25.5536, 16.9675)
  line L58 (-25.5536, 16.9675) -> (-25.753, 16.1021)
  line L59 (-25.753, 16.1021) -> (-25.0209, 15.4878)
  line L60 (-25.0209, 15.4878) -> (-24.2032, 15.8344)
  line L61 (-24.2032, 15.8344) -> (-23.4807, 16.2646)
  line L62 (-23.4807, 16.2646) -> (-22.8939, 16.7967)
  line L63 (-22.8939, 16.7967) -> (-22.2965, 17.6734)
  line L64 (-22.2965, 17.6734) -> (-21.5625, 17.2123)
  line L65 (-21.5625, 17.2123) -> (-20.7962, 16.8071)
  line L66 (-20.7962, 16.8071) -> (-21.2566, 15.8514)
  line L67 (-21.2566, 15.8514) -> (-21.4241, 15.0773)
  line L68 (-21.4241, 15.0773) -> (-21.4354, 14.2364)
  line L69 (-21.4354, 14.2364) -> (-21.3267, 13.355)
  line L70 (-21.3267, 13.355) -> (-20.4287, 13.0281)
  line L71 (-20.4287, 13.0281) -> (-19.7789, 13.6335)
  line L72 (-19.7789, 13.6335) -> (-19.2471, 14.2849)
  line L73 (-19.2471, 14.2849) -> (-18.8777, 14.9856)
  line L74 (-18.8777, 14.9856) -> (-18.6161, 16.0137)
  line L75 (-18.6161, 16.0137) -> (-17.7687, 15.8314)
  line L76 (-17.7687, 15.8314) -> (-16.91, 15.7128)
  line L77 (-16.91, 15.7128) -> (-17.0158, 14.6573)
  line L78 (-17.0158, 14.6573) -> (-16.9084, 13.8725)
  line L79 (-16.9084, 13.8725) -> (-16.6314, 13.0785)
  line L80 (-16.6314, 13.0785) -> (-16.2278, 12.2874)
  line L81 (-16.2278, 12.2874) -> (-15.2722, 12.2874)
  line L82 (-15.2722, 12.2874) -> (-14.8686, 13.0785)
  line L83 (-14.8686, 13.0785) -> (-14.5916, 13.8725)
  line L84 (-14.5916, 13.8725) -> (-14.4842, 14.6573)
  line L85 (-14.4842, 14.6573) -> (-14.59, 15.7128)
  line L86 (-14.59, 15.7128) -> (-13.7313, 15.8314)
  line L87 (-13.7313, 15.8314) -> (-12.8839, 16.0137)
  line L88 (-12.8839, 16.0137) -> (-12.6223, 14.9856)
  line L89 (-12.6223, 14.9856) -> (-12.2529, 14.2849)
  line L90 (-12.2529, 14.2849) -> (-11.7211, 13.6335)
  line L91 (-11.7211, 13.6335) -> (-11.0713, 13.0281)
  line L92 (-11.0713, 13.0281) -> (-10.1733, 13.355)
  line L93 (-10.1733, 13.355) -> (-10.0646, 14.2364)
  line L94 (-10.0646, 14.2364) -> (-10.0759, 15.0773)
  line L95 (-10.0759, 15.0773) -> (-10.2434, 15.8514)
  line L96 (-10.2434, 15.8514) -> (-10.7038, 16.8071)
  line L97 (-10.7038, 16.8071) -> (-9.9375, 17.2123)
  line L98 (-9.9375, 17.2123) -> (-9.2035, 17.6734)
  line L99 (-9.2035, 17.6734) -> (-8.6061, 16.7967)
  line L100 (-8.6061, 16.7967) -> (-8.0193, 16.2646)
  line L101 (-8.0193, 16.2646) -> (-7.2968, 15.8344)
  line L102 (-7.2968, 15.8344) -> (-6.4791, 15.4878)
  line L103 (-6.4791, 15.4878) -> (-5.747, 16.1021)
  line L104 (-5.747, 16.1021) -> (-5.9464, 16.9675)
  line L105 (-5.9464, 16.9675) -> (-6.2446, 17.7538)
  line L106 (-6.2446, 17.7538) -> (-6.6667, 18.424)
  line L107 (-6.6667, 18.424) -> (-7.4263, 19.1646)
  line L108 (-7.4263, 19.1646) -> (-6.8447, 19.8074)
  line L109 (-6.8447, 19.8074) -> (-6.3127, 20.4917)
  line L110 (-6.3127, 20.4917) -> (-5.4515, 19.8723)
  line L111 (-5.4515, 19.8723) -> (-4.7181, 19.573)
  line L112 (-4.7181, 19.573) -> (-3.892, 19.4158)
  line L113 (-3.892, 19.4158) -> (-3.0051, 19.3698)
  line L114 (-3.0051, 19.3698) -> (-2.5273, 20.1974)
  line L115 (-2.5273, 20.1974) -> (-3.0106, 20.9425)
  line L116 (-3.0106, 20.9425) -> (-3.5598, 21.5793)
  line L117 (-3.5598, 21.5793) -> (-4.1856, 22.0648)
  line L118 (-4.1856, 22.0648) -> (-5.1527, 22.5009)
  line L119 (-5.1527, 22.5009) -> (-4.8261, 23.3038)
  line L120 (-4.8261, 23.3038) -> (-4.5602, 24.1289)
  line L121 (-4.5602, 24.1289) -> (-3.539, 23.8413)
  line L122 (-3.539, 23.8413) -> (-2.7475, 23.8109)
  line L123 (-2.7475, 23.8109) -> (-1.9175, 23.9458)
  line L124 (-1.9175, 23.9458) -> (-1.0684, 24.2058)
  line L125 (-1.0684, 24.2058) -> (-0.9024, 25.147)
  line L126 (-0.9024, 25.147) -> (-1.6114, 25.6818)
  line L127 (-1.6114, 25.6818) -> (-2.3453, 26.0924)
  line L128 (-2.3453, 26.0924) -> (-3.0994, 26.3345)
  line L129 (-3.0994, 26.3345) -> (-4.1573, 26.4136)
  line L130 (-4.1573, 26.4136) -> (-4.125, 27.2798)
  line L131 (-4.125, 27.2798) -> (-4.1573, 28.146)
  line L132 (-4.1573, 28.146) -> (-3.0994, 28.2251)
  line L133 (-3.0994, 28.2251) -> (-2.3453, 28.4672)
  line L134 (-2.3453, 28.4672) -> (-1.6114, 28.8778)
  line L135 (-1.6114, 28.8778) -> (-0.9024, 29.4126)
  line L136 (-0.9024, 29.4126) -> (-1.0684, 30.3538)
  line L137 (-1.0684, 30.3538) -> (-1.9175, 30.6138)
  line L138 (-1.9175, 30.6138) -> (-2.7475, 30.7487)
  line L139 (-2.7475, 30.7487) -> (-3.539, 30.7183)
  line L140 (-3.539, 30.7183) -> (-4.5602, 30.4307)
  line L141 (-4.5602, 30.4307) -> (-4.8261, 31.2558)
  line L142 (-4.8261, 31.2558) -> (-5.1527, 32.0587)
  line L143 (-5.1527, 32.0587) -> (-4.1856, 32.4948)
  line L144 (-4.1856, 32.4948) -> (-3.5598, 32.9803)
  line L145 (-3.5598, 32.9803) -> (-3.0106, 33.6171)
  line L146 (-3.0106, 33.6171) -> (-2.5273, 34.3622)
  line L147 (-2.5273, 34.3622) -> (-3.0051, 35.1898)
  line L148 (-3.0051, 35.1898) -> (-3.892, 35.1438)
  line L149 (-3.892, 35.1438) -> (-4.7181, 34.9866)
  line L150 (-4.7181, 34.9866) -> (-5.4515, 34.6873)
  line L151 (-5.4515, 34.6873) -> (-6.3127, 34.0679)
  line L152 (-6.3127, 34.0679) -> (-6.8447, 34.7522)
  line L153 (-6.8447, 34.7522) -> (-7.4263, 35.395)
  line L154 (-7.4263, 35.395) -> (-6.6667, 36.1356)
  line L155 (-6.6667, 36.1356) -> (-6.2446, 36.8058)
  line L156 (-6.2446, 36.8058) -> (-5.9464, 37.5921)
  line L157 (-5.9464, 37.5921) -> (-5.747, 38.4575)
  line L158 (-5.747, 38.4575) -> (-6.4791, 39.0718)
  line L159 (-6.4791, 39.0718) -> (-7.2968, 38.7252)
  line L160 (-7.2968, 38.7252) -> (-8.0193, 38.295)
  line L161 (-8.0193, 38.295) -> (-8.6061, 37.7629)
  line L162 (-8.6061, 37.7629) -> (-9.2035, 36.8862)
  line L163 (-9.2035, 36.8862) -> (-9.9375, 37.3473)
  line L164 (-9.9375, 37.3473) -> (-10.7038, 37.7525)
  line L165 (-10.7038, 37.7525) -> (-10.2434, 38.7082)
  line L166 (-10.2434, 38.7082) -> (-10.0759, 39.4823)
  line L167 (-10.0759, 39.4823) -> (-10.0646, 40.3232)
  line L168 (-10.0646, 40.3232) -> (-10.1733, 41.2046)
  line L169 (-10.1733, 41.2046) -> (-11.0713, 41.5315)
  line L170 (-11.0713, 41.5315) -> (-11.7211, 40.9261)
  line L171 (-11.7211, 40.9261) -> (-12.2529, 40.2747)
  line L172 (-12.2529, 40.2747) -> (-12.6223, 39.574)
  line L173 (-12.6223, 39.574) -> (-12.8839, 38.5459)
  line L174 (-12.8839, 38.5459) -> (-13.7313, 38.7282)
  line L175 (-13.7313, 38.7282) -> (-14.59, 38.8468)
  line L176 (-14.59, 38.8468) -> (-14.4842, 39.9023)
  line L177 (-14.4842, 39.9023) -> (-14.5916, 40.6871)
  line L178 (-14.5916, 40.6871) -> (-14.8686, 41.4811)
  line L179 (-14.8686, 41.4811) -> (-15.2722, 42.2722)
  line L180 (-15.2722, 42.2722) -> (-16.2278, 42.2722)
  line L181 (-16.2278, 42.2722) -> (-16.6314, 41.4811)
  line L182 (-16.6314, 41.4811) -> (-16.9084, 40.6871)
  line L183 (-16.9084, 40.6871) -> (-17.0158, 39.9023)
  line L184 (-17.0158, 39.9023) -> (-16.91, 38.8468)
  line L185 (-16.91, 38.8468) -> (-17.7687, 38.7282)
  line L186 (-17.7687, 38.7282) -> (-18.6161, 38.5459)
  line L187 (-18.6161, 38.5459) -> (-18.8777, 39.574)
  line L188 (-18.8777, 39.574) -> (-19.2471, 40.2747)
  line L189 (-19.2471, 40.2747) -> (-19.7789, 40.9261)
  line L190 (-19.7789, 40.9261) -> (-20.4287, 41.5315)
  line L191 (-20.4287, 41.5315) -> (-21.3267, 41.2046)
  line L192 (-21.3267, 41.2046) -> (-21.4354, 40.3232)
  line L193 (-21.4354, 40.3232) -> (-21.4241, 39.4823)
  line L194 (-21.4241, 39.4823) -> (-21.2566, 38.7082)
  line L195 (-21.2566, 38.7082) -> (-20.7962, 37.7525)
  line L196 (-20.7962, 37.7525) -> (-21.5625, 37.3473)
  line L197 (-21.5625, 37.3473) -> (-22.2965, 36.8862)
extrude "Stage1_Planet_B_Extrude" add sketch "スケッチ1 (5)" along normal blind 12 from surface at 34 separate body makes body 5 in component "Stage1_Planet_Gear_B"
sketch "スケッチ2 (5)" plane through (0, 0, 0) normal (0, 0, 1) x (1, 0, 0) in component "Stage1_Planet_Gear_B"
  circle A0 centre (-15.75, 27.2798) radius 8
extrude "Stage1_Planet_B_Hub_Lower_Extrude" add sketch "スケッチ2 (5)" along normal blind 3.5 from surface at 30.5 bodies 5 in component "Stage1_Planet_Gear_B"
sketch "スケッチ3 (5)" plane through (0, 0, 0) normal (0, 0, 1) x (1, 0, 0) in component "Stage1_Planet_Gear_B"
  circle A0 centre (-15.75, 27.2798) radius 8
extrude "Stage1_Planet_B_Hub_Upper_Extrude" add sketch "スケッチ3 (5)" along normal blind 3.5 from surface at 46 bodies 5 in component "Stage1_Planet_Gear_B"
sketch "スケッチ4 (5)" plane through (0, 0, 0) normal (0, 0, 1) x (1, 0, 0) in component "Stage1_Planet_Gear_B"
  circle A0 centre (-15.75, 27.2798) radius 4.3
extrude "Stage1_Planet_B_Bore_Cut" cut sketch "スケッチ4 (5)" along normal blind 22 from surface at 29 bodies 5 in component "Stage1_Planet_Gear_B"